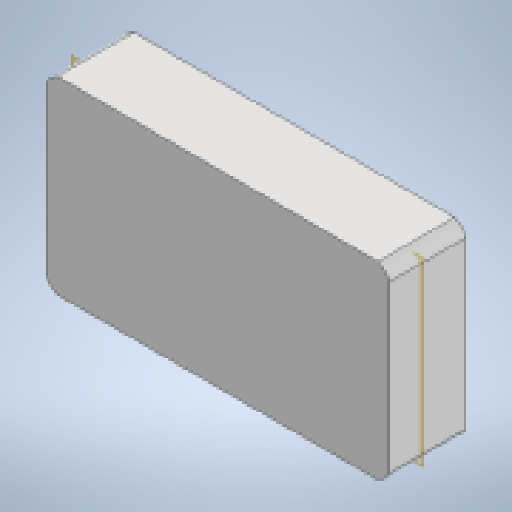
# Autodesk Inventor part: Housing Bottom
Saved by Autodesk Inventor 2023 (Build 270158000, 158)
## iProperties
Created: 2023-06-04
Part Number: Housing Bottom
Material: Generic
Document SubType Name: Modeling
Designer: jeffb
Density: 1 g/cm^3
Appearance: Default
Author: jeffb
Autodesk Inventor part; units mm, degrees
ref_plane "YZ Plane" through (0, 0, 0) normal (1, 0, 0) x (0, 1, 0)
ref_plane "XZ Plane" through (0, 0, 0) normal (0, 1, 0) x (-1, 0, 0)
ref_plane "XY Plane" through (0, 0, 0) normal (0, 0, 1) x (1, 0, 0)
ref_plane "Work Plane1" through (0, 0, 0) normal (0, 0, 1) x (1, 0, 0)
sketch "Sketch1" plane through (0, 0, 0) normal (0, 0, 1) x (1, 0, 0)
  circle A0 centre (48.5, 23.5) radius 1.6 construction
  circle A1 centre (48.5, -23.5) radius 1.6 construction
  circle A2 centre (-48.5, -23.5) radius 1.6 construction
  circle A3 centre (-48.5, 23.5) radius 1.6 construction
  circle A4 centre (48.5, 23.5) radius 1.2192
  circle A5 centre (48.5, -23.5) radius 1.2192
  circle A6 centre (-48.5, -23.5) radius 1.2192
  circle A7 centre (-48.5, 23.5) radius 1.2192
  circle A8 centre (48.5, 23.5) radius 3.7192
  arc A9 (46.3017, -26.5) -> (45.3587, -21.5088) centre (48.5, -23.5) ccw
  circle A10 centre (-48.5, 23.5) radius 3.7192
  arc A11 (-45.3587, -21.5088) -> (-46.3017, -26.5) centre (-48.5, -23.5) ccw
  line L0 (51.5, -26.5) -> (51.5, 26.5) projected
  line L1 (51.5, 26.5) -> (-51.5, 26.5) projected
  line L2 (-51.5, -26.5) -> (51.5, -26.5) projected
  line L3 (-51.5, 26.5) -> (-51.5, -26.5) projected
  line L4 (-51.5, -26.5) -> (51.5, -26.5) construction
  line L5 (51.5, -26.5) -> (51.5, 26.5) construction
  line L6 (51.5, 26.5) -> (-51.5, 26.5) construction
  line L7 (-51.5, 26.5) -> (-51.5, -26.5) construction
  circle A12 centre (-48.5, -23.5) radius 1.6 construction
  circle A13 centre (-27.0556, -20.7948) radius 0.35 construction
  circle A14 centre (-25.0556, -20.7948) radius 0.35 construction
  circle A15 centre (-43.5468, -18.5088) radius 0.505 construction
  circle A16 centre (-41.0068, -18.5088) radius 0.505 construction
  circle A17 centre (-38.4668, -18.5088) radius 0.505 construction
  circle A18 centre (-43.5468, -13.4288) radius 0.605 construction
  circle A19 centre (-41.0068, -13.4288) radius 0.605 construction
  circle A20 centre (-38.4668, -13.4288) radius 0.605 construction
  circle A21 centre (-35.9268, -18.5088) radius 0.505 construction
  circle A22 centre (-35.9268, -13.4288) radius 0.605 construction
  circle A23 centre (-23.0556, -20.7948) radius 0.35 construction
  circle A24 centre (-21.0556, -20.7948) radius 0.35 construction
  circle A25 centre (-10.0696, -17.2388) radius 0.5 construction
  circle A26 centre (-7.5296, -17.2388) radius 0.5 construction
  circle A27 centre (-4.9896, -17.2388) radius 0.5 construction
  circle A28 centre (-46.9416, -1.9508) radius 0.35 construction
  circle A29 centre (-38.0516, -1.9508) radius 0.35 construction
  circle A30 centre (-24.8016, -11.6508) radius 0.4826 construction
  circle A31 centre (-22.2616, -11.6508) radius 0.4826 construction
  circle A32 centre (-19.7216, -11.6508) radius 0.4826 construction
  circle A33 centre (-17.1816, -11.6508) radius 0.4826 construction
  circle A34 centre (-14.6416, -11.6508) radius 0.4826 construction
  circle A35 centre (-24.8016, -9.1108) radius 0.4826 construction
  circle A36 centre (-24.8016, -6.5708) radius 0.4826 construction
  circle A37 centre (-12.1016, -11.6508) radius 0.4826 construction
  circle A38 centre (-9.5616, -11.6508) radius 0.4826 construction
  circle A39 centre (-9.5616, -9.1108) radius 0.4826 construction
  circle A40 centre (-9.5616, -6.5708) radius 0.4826 construction
  circle A41 centre (-24.8016, -4.0308) radius 0.4826 construction
  circle A42 centre (-24.8016, -1.4908) radius 0.4826 construction
  circle A43 centre (-9.5616, -4.0308) radius 0.4826 construction
  circle A44 centre (-9.5616, -1.4908) radius 0.4826 construction
  circle A45 centre (1.6144, -18.5088) radius 0.505 construction
  circle A46 centre (4.1544, -18.5088) radius 0.505 construction
  circle A47 centre (6.6944, -18.5088) radius 0.505 construction
  circle A48 centre (9.2344, -18.5088) radius 0.505 construction
  circle A49 centre (1.6144, -13.4288) radius 0.605 construction
  circle A50 centre (4.1544, -13.4288) radius 0.605 construction
  circle A51 centre (6.6944, -13.4288) radius 0.605 construction
  circle A52 centre (9.2344, -13.4288) radius 0.605 construction
  circle A53 centre (17.1084, -18.5088) radius 0.505 construction
  circle A54 centre (19.6484, -18.5088) radius 0.505 construction
  circle A55 centre (22.1884, -18.5088) radius 0.505 construction
  circle A56 centre (24.7284, -18.5088) radius 0.505 construction
  circle A57 centre (17.1084, -13.4288) radius 0.605 construction
  circle A58 centre (19.6484, -13.4288) radius 0.605 construction
  circle A59 centre (22.1884, -13.4288) radius 0.605 construction
  circle A60 centre (24.7284, -13.4288) radius 0.605 construction
  circle A61 centre (48.5, -23.5) radius 1.6 construction
  circle A62 centre (32.3484, -18.5088) radius 0.505 construction
  circle A63 centre (34.8884, -18.5088) radius 0.505 construction
  circle A64 centre (37.4284, -18.5088) radius 0.505 construction
  circle A65 centre (32.3484, -13.4288) radius 0.605 construction
  circle A66 centre (34.8884, -13.4288) radius 0.605 construction
  circle A67 centre (37.4284, -13.4288) radius 0.605 construction
  circle A68 centre (39.9684, -18.5088) radius 0.505 construction
  circle A69 centre (39.9684, -13.4288) radius 0.605 construction
  circle A70 centre (-46.9416, 0.0492) radius 0.35 construction
  circle A71 centre (-46.9416, 2.0492) radius 0.35 construction
  circle A72 centre (-38.0516, 0.0492) radius 0.35 construction
  circle A73 centre (-38.0516, 2.0492) radius 0.35 construction
  circle A74 centre (-46.9416, 4.0492) radius 0.35 construction
  circle A75 centre (-38.0516, 4.0492) radius 0.35 construction
  circle A76 centre (-46.9416, 11.7492) radius 0.35 construction
  circle A77 centre (-38.0516, 12.0192) radius 0.35 construction
  circle A78 centre (-24.8016, 1.0492) radius 0.4826 construction
  circle A79 centre (-24.8016, 3.5892) radius 0.4826 construction
  circle A80 centre (-24.8016, 6.1292) radius 0.4826 construction
  circle A81 centre (-9.5616, 1.0492) radius 0.4826 construction
  circle A82 centre (-9.5616, 3.5892) radius 0.4826 construction
  circle A83 centre (-9.5616, 6.1292) radius 0.4826 construction
  circle A84 centre (-24.8016, 8.6692) radius 0.4826 construction
  circle A85 centre (-24.8016, 11.2092) radius 0.4826 construction
  circle A86 centre (-9.5616, 8.6692) radius 0.4826 construction
  circle A87 centre (-9.5616, 11.2092) radius 0.4826 construction
  circle A88 centre (-46.9416, 13.7492) radius 0.35 construction
  circle A89 centre (-38.0516, 14.0192) radius 0.35 construction
  circle A90 centre (-46.9416, 15.7492) radius 0.35 construction
  circle A91 centre (-46.9416, 17.7492) radius 0.35 construction
  circle A92 centre (-38.0516, 16.0192) radius 0.35 construction
  circle A93 centre (-38.0516, 18.0192) radius 0.35 construction
  circle A94 centre (-48.5, 23.5) radius 1.6 construction
  circle A95 centre (-24.8016, 13.7492) radius 0.4826 construction
  circle A96 centre (-24.8016, 16.2892) radius 0.4826 construction
  circle A97 centre (-9.5616, 13.7492) radius 0.4826 construction
  circle A98 centre (-9.5616, 16.2892) radius 0.4826 construction
  circle A99 centre (-2.9576, 18.6392) radius 0.51 construction
  circle A100 centre (-0.4176, 18.6392) radius 0.51 construction
  circle A101 centre (-24.8016, 18.8292) radius 0.4826 construction
  circle A102 centre (-24.8016, 21.3692) radius 0.4826 construction
  circle A103 centre (-9.5616, 18.8292) radius 0.4826 construction
  circle A104 centre (-9.5616, 21.3692) radius 0.4826 construction
  circle A105 centre (48.5, 23.5) radius 1.6 construction
  line L8 (-46.3017, -26.5) -> (46.3017, -26.5)
  line L9 (-30.0556, -21.5088) -> (-30.0556, -23.7948)
  line L10 (-30.0556, -23.7948) -> (-18.0556, -23.7948)
  line L11 (-18.0556, -23.7948) -> (-18.0556, -21.5088)
  line L12 (45.3587, -21.5088) -> (-18.0556, -21.5088)
  line L13 (-30.0556, -21.5088) -> (-45.3587, -21.5088)
  line L14 (-14.6816, 21.3692) -> (-19.6816, 21.3692)
  line L15 (-19.6816, 21.3692) -> (-19.6816, -8.6508)
  line L16 (-19.6816, -8.6508) -> (-14.6816, -8.6508)
  line L17 (-14.6816, -8.6508) -> (-14.6816, 21.3692)
  line L18 (-41.0516, 18.0192) -> (-43.9416, 18.0192)
  line L19 (-43.9416, 18.0192) -> (-43.9416, -1.9508)
  line L20 (-43.9416, -1.9508) -> (-41.0516, -1.9508)
  line L21 (-41.0516, -1.9508) -> (-41.0516, 18.0192)
  line L22 (-38.0516, -1.9508) -> (-46.9416, -1.9508) construction
  line L23 (44.1584, -5.4288) -> (0.2644, -5.4288)
  line L24 (0.2644, -5.4288) -> (0.2644, -10.4288)
  line L25 (0.2644, -10.4288) -> (44.1584, -10.4288)
  line L26 (44.1584, -10.4288) -> (44.1584, -5.4288)
  line L27 (44.1584, -11.9688) -> (44.1584, -10.4688) construction
  line L28 (0.2644, -11.9688) -> (0.2644, -10.4688) construction
  point P0 (0, 0)
  point P1 (-51.5, 25.6983)
  point P2 (-51.5, 21.3017)
  point P3 (-46.3017, 26.5)
  point P4 (-50.6983, 26.5)
  point P5 (-51.5, -21.3017)
  point P6 (-51.5, -25.6983)
  point P7 (-50.6983, -26.5)
  point P8 (-46.3017, -26.5)
  point P9 (50.6983, -26.5)
  point P10 (51.5, -25.6983)
  point P11 (51.5, -21.3017)
  point P12 (50.6983, 26.5)
  point P13 (46.3017, 26.5)
  point P14 (51.5, 21.3017)
  point P15 (51.5, 25.6983)
  point P16 (-17.1816, -8.6508)
  point P17 (-42.4966, -1.9508)
  point P18 (31.455, -21.5088)
  point P19 (40.0794, -26.5)
  point P20 (40.0794, -21.5088)
  dimension "d0" = 2.4384
  dimension "d1" = 2.5
  dimension "d6" = 3
  dimension "d7" = 3
  dimension "d8" = 3
  dimension "d9" = 48.0088
  dimension "d10" = 48.0088
  dimension "d12" = 0.8017
  dimension "d13" = 0
  dimension "d14" = 5.1983
  dimension "d15" = 0
  dimension "d16" = 47.8017
  dimension "d17" = 0
  dimension "d18" = 52.1983
  dimension "d19" = 0
  dimension "d20" = 0
  dimension "d21" = 0.8017
  dimension "d22" = 53
  dimension "d23" = 0.8017
  dimension "d24" = 0
  dimension "d25" = 5.1983
  dimension "d26" = 53
  dimension "d27" = 5.1983
  dimension "d28" = 0
  dimension "d29" = 97.8017
  dimension "d30" = 53
  dimension "d31" = 97.8017
  dimension "d32" = 0
  dimension "d33" = 102.1983
  dimension "d34" = 53
  dimension "d35" = 102.1983
  dimension "d36" = 0.8017
  dimension "d37" = 103
  dimension "d38" = 5.1983
  dimension "d39" = 103
  dimension "d40" = 47.8017
  dimension "d41" = 103
  dimension "d42" = 52.1983
  dimension "d43" = 103
  dimension "d44" = 5
  dimension "d45" = 3
  dimension "d47" = 3
  dimension "d48" = 3
  dimension "d49" = 5
  constraints: 38 end point, 11 parallel, 8 centre point, 8 coincident, 6 equal radius, 6 horizontal, 4 point on circle, 3 collinear, 3 horizontal alignment, 3 midpoint, 3 perpendicular, 2 point on line, 1 vertical alignment
  measures "d0" diameter of A5
  measures "d1" radial gap between concentric circles of A8 A4
  measures "d6" distance from line of L10 A24.centre
  measures "d7" distance from line of L11 A24.centre
  measures "d8" distance from line of A13.centre L9
  measures "d9" distance between parallel lines of L1 L12
  measures "d10" distance between parallel lines of L1 L13
  measures "d12" distance from line of point (51.5, 25.698) L6
  measures "d13" distance from line of point (51.5, 25.698) L0
  measures "d14" distance from line of point (51.5, 21.302) L6
  measures "d15" distance from line of point (51.5, 21.302) L0
  measures "d16" distance from line of point (51.5, -21.302) L6
  measures "d17" distance from line of point (51.5, -21.302) L0
  measures "d18" distance from line of point (51.5, -25.698) L6
  measures "d19" distance from line of point (51.5, -25.698) L0
  measures "d20" distance from line of point (50.698, 26.5) L6
  measures "d21" distance from line of point (50.698, 26.5) L0
  measures "d22" distance from line of point (50.698, -26.5) L6
  measures "d23" distance from line of point (50.698, -26.5) L0
  measures "d24" distance from line of point (46.302, 26.5) L6
  measures "d25" distance from line of point (46.302, 26.5) L0
  measures "d26" distance from line of point (46.302, -26.5) L6
  measures "d27" distance from line of point (46.302, -26.5) L0
  measures "d28" distance from line of point (-46.302, 26.5) L6
  measures "d29" distance from line of point (-46.302, 26.5) L0
  measures "d30" distance from line of point (-46.302, -26.5) L6
  measures "d31" distance from line of point (-46.302, -26.5) L0
  measures "d32" distance from line of point (-50.698, 26.5) L6
  measures "d33" distance from line of point (-50.698, 26.5) L0
  measures "d34" distance from line of point (-50.698, -26.5) L6
  measures "d35" distance from line of point (-50.698, -26.5) L0
  measures "d36" distance from line of point (-51.5, 25.698) L6
  measures "d37" distance from line of point (-51.5, 25.698) L0
  measures "d38" distance from line of point (-51.5, 21.302) L6
  measures "d39" distance from line of point (-51.5, 21.302) L0
  measures "d40" distance from line of point (-51.5, -21.302) L6
  measures "d41" distance from line of point (-51.5, -21.302) L0
  measures "d42" distance from line of point (-51.5, -25.698) L6
  measures "d43" distance from line of point (-51.5, -25.698) L0
  measures "d44" distance of L14.start L14.end
  measures "d45" distance from line of A33.centre L16
  measures "d47" distance from line of L21 A89.centre
  measures "d48" distance from line of A69.centre L25
  measures "d49" distance between parallel lines of L25 L23
extrude "Extrusion1" add sketch "Sketch1" along normal blind 6.35 contours L0 A8 L1 | A8 L1 L0 | L0 A9 L2 A11 L3 L13 L9 L10 L11 L12 | A10 L3 L1 | L0 L2 A9 | A10 L3 L1 | A11 L2 L3 | L17 L16 L15 L14 | L21 L20 L19 L18 | L26 L25 L24 L23
sketch "Sketch2" plane through (0, 0, 6.35) normal (0, 0, 1) x (1, 0, 0)
  line L0 (51.5, 21.3017) -> (51.5, 26.5)
  line L1 (51.5, 26.5) -> (46.3017, 26.5)
  line L2 (-51.5, -21.3017) -> (-51.5, -26.5)
  line L3 (-51.5, -26.5) -> (51.5, -26.5)
  line L4 (51.5, -26.5) -> (51.5, -21.3017)
  circle A0 centre (48.5, -23.5) radius 1.2192
  line L5 (-46.3017, 26.5) -> (-51.5, 26.5)
  line L6 (-51.5, 26.5) -> (-51.5, 21.3017)
  line L7 (-51.5, 21.3017) -> (-51.5, -21.3017)
  line L8 (-46.3017, 26.5) -> (46.3017, 26.5)
  arc A1 (51.5, -21.3017) -> (45.3587, -21.5088) centre (48.5, -23.5) ccw projected
  line L9 (51.5, 21.3017) -> (51.5, -21.3017)
  line L10 (-51.5, -26.5) -> (51.5, -26.5)
  line L11 (51.5, -26.5) -> (51.5, -21.3017)
  line L12 (-46.3017, 26.5) -> (-51.5, 26.5)
  line L13 (-51.5, 26.5) -> (-51.5, 21.3017)
  line L14 (-51.5, -26.5) -> (51.5, -26.5)
  arc A2 (-51.5, 21.3017) -> (-46.3017, 26.5) centre (-48.5, 23.5) ccw
  arc A3 (46.3017, 26.5) -> (51.5, 21.3017) centre (48.5, 23.5) ccw
  line L15 (51.5, 21.3017) -> (51.5, 26.5)
  line L16 (51.5, 26.5) -> (46.3017, 26.5)
  arc A4 (-45.3587, -21.5088) -> (-51.5, -21.3017) centre (-48.5, -23.5) ccw
  line L17 (-51.5, -21.3017) -> (-51.5, -26.5)
  arc A5 (51.5, -21.3017) -> (45.3587, -21.5088) centre (48.5, -23.5) ccw
  line L18 (45.3587, -21.5088) -> (-18.0556, -21.5088)
  line L19 (-18.0556, -21.5088) -> (-18.0556, -23.7948)
  line L20 (-18.0556, -23.7948) -> (-30.0556, -23.7948)
  line L21 (-30.0556, -23.7948) -> (-30.0556, -21.5088)
  line L22 (-30.0556, -21.5088) -> (-45.3587, -21.5088)
  arc A6 (-51.5, 21.3017) -> (-46.3017, 26.5) centre (-48.5, 23.5) ccw
  line L23 (-51.5, 26.5) -> (-51.5, 21.3017)
  arc A7 (46.3017, 26.5) -> (51.5, 21.3017) centre (48.5, 23.5) ccw
  line L24 (51.5, 21.3017) -> (51.5, 26.5)
  line L25 (51.5, 26.5) -> (46.3017, 26.5)
  arc A8 (-45.3587, -21.5088) -> (-51.5, -21.3017) centre (-48.5, -23.5) ccw
  arc A9 (51.5, -21.3017) -> (45.3587, -21.5088) centre (48.5, -23.5) ccw
  line L26 (45.3587, -21.5088) -> (-18.0556, -21.5088)
  line L27 (-18.0556, -21.5088) -> (-18.0556, -23.7948)
  line L28 (-18.0556, -23.7948) -> (-30.0556, -23.7948)
  line L29 (-30.0556, -23.7948) -> (-30.0556, -21.5088)
  line L30 (-30.0556, -21.5088) -> (-45.3587, -21.5088)
  arc A10 (-51.5, 21.3017) -> (-46.3017, 26.5) centre (-48.5, 23.5) ccw
  line L31 (-46.3017, 26.5) -> (-51.5, 26.5)
  arc A11 (46.3017, 26.5) -> (51.5, 21.3017) centre (48.5, 23.5) ccw
  arc A12 (-45.3587, -21.5088) -> (-51.5, -21.3017) centre (-48.5, -23.5) ccw
  line L32 (-51.5, -21.3017) -> (-51.5, -26.5)
  line L33 (51.5, -26.5) -> (51.5, -21.3017)
  arc A13 (51.5, -21.3017) -> (45.3587, -21.5088) centre (48.5, -23.5) ccw
  line L34 (45.3587, -21.5088) -> (-18.0556, -21.5088)
  line L35 (-18.0556, -21.5088) -> (-18.0556, -23.7948)
  line L36 (-18.0556, -23.7948) -> (-30.0556, -23.7948)
  line L37 (-30.0556, -23.7948) -> (-30.0556, -21.5088)
  line L38 (-30.0556, -21.5088) -> (-45.3587, -21.5088)
  point P0 (0, 0)
  point P1 (-51.5, -26.5)
  point P2 (45.3587, -21.5088)
  dimension "d58" = 3.7192
  dimension "d59" = 3.7192
  dimension "d60" = 3.7192
  dimension "d61" = 3.7192
  dimension "d62" = 3.7192
  dimension "d63" = 2.4384
  dimension "d64" = 3.7192
  dimension "d65" = 3.7192
  dimension "d66" = 3.7192
  dimension "d67" = 3.7192
  dimension "d68" = 90
  dimension "d69" = 90
  dimension "d70" = 90
  dimension "d71" = 90
  dimension "d72" = 90
  dimension "d73" = 90
  dimension "d74" = 90
  dimension "d75" = 90
  dimension "d76" = 90
  dimension "d77" = 90
  dimension "d78" = 90
  dimension "d79" = 90
  dimension "d80" = 90
  dimension "d81" = 90
  dimension "d82" = 90
  dimension "d83" = 90
  dimension "d84" = 90
  dimension "d85" = 90
  dimension "d86" = 90
  dimension "d87" = 90
  dimension "d88" = 90
  dimension "d89" = 90
  dimension "d90" = 90
  dimension "d91" = 90
  dimension "d92" = 90
  dimension "d93" = 90
  dimension "d94" = 90
  dimension "d95" = 90
  dimension "d96" = 90
  dimension "d97" = 69.5556
  dimension "d98" = 81.5556
  dimension "d99" = 103
  dimension "d100" = 103
  dimension "d101" = 48.0088
  dimension "d102" = 2.286
  dimension "d103" = 48.0088
  dimension "d104" = 4.9912
  dimension "d105" = 47.8017
  dimension "d106" = 47.8017
  dimension "d107" = 47.8017
  dimension "d108" = 0
  dimension "d109" = 0
  dimension "d110" = 0
  dimension "d111" = 0
  dimension "d112" = 0
  dimension "d113" = 0
  dimension "d114" = 0.2071
  dimension "d115" = 0.2071
  dimension "d116" = 0.2071
  dimension "d117" = 69.5556
  dimension "d118" = 69.5556
  dimension "d119" = 2.4931
  dimension "d120" = 2.4931
  dimension "d121" = 0.2071
  constraints: 78 end point, 24 point on circle, 13 centre point, 6 parallel, 3 equal radius, 2 vertical, 1 concentric, 1 horizontal, 1 perpendicular
  measures "d58" radius of A11
  measures "d59" radius of A7
  measures "d60" radius of A13
  measures "d61" radius of A9
  measures "d62" radius of A5
  measures "d63" diameter of A0
  measures "d64" radius of A10
  measures "d65" radius of A6
  measures "d66" radius of A12
  measures "d67" radius of A8
  measures "d68" angle of L1 L0
  measures "d69" angle of L1 L24
  measures "d70" angle of L1 L15
  measures "d71" angle of L9 L1
  measures "d72" angle of L1 L33
  measures "d73" angle of L1 L4
  measures "d74" angle of L1 L11
  measures "d75" angle of L1 L35
  measures "d76" angle of L1 L27
  measures "d77" angle of L1 L37
  measures "d78" angle of L1 L29
  measures "d79" angle of L1 L13
  measures "d80" angle of L1 L23
  measures "d81" angle of L1 L32
  measures "d82" angle of L1 L2
  measures "d83" angle of L1 L17
  measures "d84" angle of L0 L25
  measures "d85" angle of L0 L16
  measures "d86" angle of L0 L34
  measures "d87" angle of L0 L26
  measures "d88" angle of L0 L36
  measures "d89" angle of L0 L28
  measures "d90" angle of L0 L38
  measures "d91" angle of L0 L30
  measures "d92" angle of L0 L22
  measures "d93" angle of L0 L31
  measures "d94" angle of L0 L12
  measures "d95" angle of L0 L14
  measures "d96" angle of L0 L3
  measures "d97" distance between parallel lines of L15 L19
  measures "d98" distance between parallel lines of L15 L21
  measures "d99" distance between parallel lines of L15 L6
  measures "d100" distance between parallel lines of L7 L15
  measures "d101" distance between parallel lines of L8 L18
  measures "d102" distance between parallel lines of L18 L20
  measures "d103" distance between parallel lines of L18 L5
  measures "d104" distance between parallel lines of L18 L10
  measures "d105" distance from line of L9.end L1
  measures "d106" distance from line of L9.end L25
  measures "d107" distance from line of L9.end L16
  measures "d108" distance from line of L9.end L0
  measures "d109" distance from line of L9.end L24
  measures "d110" distance from line of L9.end L15
  measures "d111" distance from line of L9.end L33
  measures "d112" distance from line of L9.end L4
  measures "d113" distance from line of L9.end L11
  measures "d114" distance from line of L9.end L34
  measures "d115" distance from line of L9.end L26
  measures "d116" distance from line of L9.end L18
  measures "d117" distance from line of L9.end L35
  measures "d118" distance from line of L9.end L27
  measures "d119" distance from line of L9.end L36
  measures "d120" distance from line of L9.end L28
  measures "d121" distance from line of L9.end L38
extrude "Extrusion2" add sketch "Sketch2" along normal blind 3.175 contours A3 L1 L0 | L9 A1 L18 L19 L20 L21 L22 A4 L7 A2 L8 A3 | L4 L3 L2 A4 L22 L21 L20 L19 L18 A1 | A2 L6 L5 | A0
sketch "Sketch3" plane through (0, 0, 9.525) normal (0, 0, 1) x (1, 0, 0)
  circle A0 centre (48.5, -23.5) radius 1.2192 projected
  arc A1 (-53.5, -26.2766) -> (-51.2766, -28.5) centre (-48.5, -23.5) ccw
  line L0 (-51.2766, -28.5) -> (51.2766, -28.5)
  arc A2 (51.2766, -28.5) -> (53.5, -26.2766) centre (48.5, -23.5) ccw
  line L1 (53.5, -26.2766) -> (53.5, 26.2766)
  arc A3 (53.5, 26.2766) -> (51.2766, 28.5) centre (48.5, 23.5) ccw
  line L2 (51.2766, 28.5) -> (-51.2766, 28.5)
  arc A4 (-51.2766, 28.5) -> (-53.5, 26.2766) centre (-48.5, 23.5) ccw
  line L3 (-53.5, 26.2766) -> (-53.5, -26.2766)
  point P0 (0, 0)
  constraints: 8 end point, 8 point on circle, 4 centre point
extrude "Extrusion3" add sketch "Sketch3" against normal up to surface (3.175 mm away) contours A0 | L3 A4 L2 A3 L1 A2 L0 A1
sketch "Sketch4" plane through (0, 0, 9.525) normal (0, 0, 1) x (1, 0, 0)
  line L0 (-55.5, -26.7536) -> (-55.5, 26.7536)
  arc A0 (-51.7536, 30.5) -> (-55.5, 26.7536) centre (-48.5, 23.5) ccw
  line L1 (-51.7536, 30.5) -> (51.7536, 30.5)
  arc A1 (55.5, 26.7536) -> (51.7536, 30.5) centre (48.5, 23.5) ccw
  line L2 (55.5, 26.7536) -> (55.5, -26.7536)
  arc A2 (51.7536, -30.5) -> (55.5, -26.7536) centre (48.5, -23.5) ccw
  line L3 (51.7536, -30.5) -> (-51.7536, -30.5)
  arc A3 (-55.5, -26.7536) -> (-51.7536, -30.5) centre (-48.5, -23.5) ccw
  line L4 (-51.2766, -28.5) -> (51.2766, -28.5) projected
  arc A4 (51.2766, -28.5) -> (53.5, -26.2766) centre (48.5, -23.5) ccw projected
  line L5 (53.5, -26.2766) -> (53.5, 26.2766) projected
  arc A5 (53.5, 26.2766) -> (51.2766, 28.5) centre (48.5, 23.5) ccw projected
  line L6 (51.2766, 28.5) -> (-51.2766, 28.5) projected
  arc A6 (-51.2766, 28.5) -> (-53.5, 26.2766) centre (-48.5, 23.5) ccw projected
  line L7 (-53.5, 26.2766) -> (-53.5, -26.2766) projected
  arc A7 (-53.5, -26.2766) -> (-51.2766, -28.5) centre (-48.5, -23.5) ccw projected
  point P0 (0, 0)
  constraints: 8 end point, 8 point on circle, 4 centre point
ref_plane "Work Plane2" through (-44.8968, -20.4688, -15.23) normal (0, 0, -1) x (0, 1, 0)
extrude "Extrusion4" add sketch "Sketch4" against normal up to surface (24.755 mm away)
body "Solid1"
